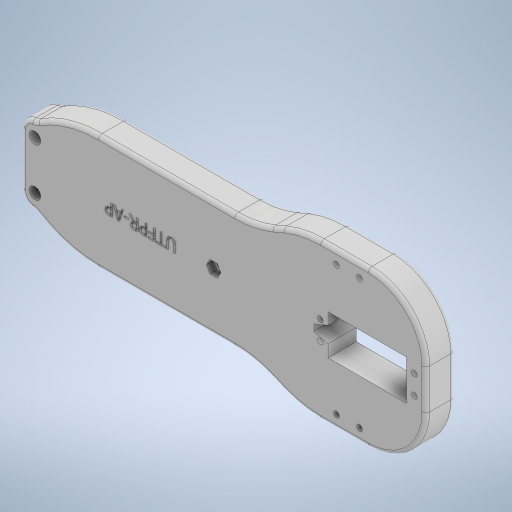
# Autodesk Inventor part: Corpo
Saved by Autodesk Inventor 2024.1 (Build 281209000, 209)
## iProperties
Created: 2024-11-07
Part Number: Corpo
Material: Genérico
Document SubType Name: Modeling
Designer: dimit
Density: 1 g/cm^3
Appearance: Padrão
Author: dimit
Autodesk Inventor part; units mm, degrees
ref_plane "YZ Plane" through (0, 0, 0) normal (1, 0, 0) x (0, 1, 0)
ref_plane "XZ Plane" through (0, 0, 0) normal (0, 1, 0) x (-1, 0, 0)
ref_plane "XY Plane" through (0, 0, 0) normal (0, 0, 1) x (1, 0, 0)
sketch "Esboço1" plane through (0, 0, 0) normal (0, 0, 1) x (1, 0, 0)
  line L0 (44.0084, -10.3855) -> (3.1399, -10.3855)
  line L1 (3.1399, -10.3855) -> (3.1399, 10.3339)
  line L2 (3.1399, 10.3339) -> (44.0084, 10.3339)
  line L3 (44.0084, 10.3339) -> (44.0084, -10.3855)
  line L4 (3.1399, -3.9571) -> (-0.3989, -3.0305)
  line L5 (-0.3989, -3.0305) -> (-1.7282, -2.0962)
  line L6 (-1.7282, -2.0962) -> (-1.7282, 2.1181)
  line L7 (-1.7282, 2.1181) -> (0.2728, 3.0795)
  line L8 (0.2728, 3.0795) -> (3.1399, 4.3343)
  arc A0 (-2.1758, -6.5758) -> (-2.0383, -3.326) centre (-0.9442, -5.0001) ccw
  circle A1 centre (-0.9442, -5.0001) radius 1.9999
  arc A2 (-1.7945, 3.19) -> (0.8219, 4.0617) centre (-0.9442, 5.0002) ccw
  circle A3 centre (-0.9442, 5.0002) radius 2
  arc A4 (46.0562, 5.0474) -> (49.3616, 3.4857) centre (48.0575, 5.0043) ccw
  circle A5 centre (48.0575, 5.0043) radius 2.0017
  arc A6 (48.3945, -3.0289) -> (46.5433, -6.3084) centre (48.0557, -4.9999) ccw
  circle A7 centre (48.0557, -4.9999) radius 1.9999
  line L9 (44.0084, -10.3855) -> (44.0084, -40.3855)
  line L10 (44.0084, 10.3339) -> (44.0084, 40.3339)
  line L11 (44.0084, 40.3339) -> (54.0084, 40.3339)
  line L12 (54.0084, 40.3339) -> (54.0084, -40.3855)
  line L13 (54.0084, -40.3855) -> (44.0084, -40.3855)
  line L14 (-105.4392, -0.0258) -> (-145.4392, -0.0258)
  line L15 (-145.4392, -0.0258) -> (-145.4392, -30.0258)
  line L16 (-145.4392, -30.0258) -> (-145.4392, 29.9742)
  line L17 (-145.4392, 29.9742) -> (-35.4392, 29.9742)
  line L18 (44.0084, 40.3339) -> (-10.9916, 40.3339)
  line L19 (-10.9916, 40.3339) -> (-35.4392, 29.9742)
  line L20 (44.0084, -40.3855) -> (-10.9916, -40.3855)
  line L21 (-145.4392, -30.0258) -> (-35.4392, -30.0258)
  line L22 (-35.4392, -30.0258) -> (-10.9916, -40.3855)
  point P0 (0, 0)
  point P1 (48.3945, -3.0289)
  point P2 (-2.1758, -6.5758)
  point P3 (-2.0383, -3.326)
  point P4 (0.8219, 4.0617)
  dimension "d0" = 2
  dimension "d1" = 30
  dimension "d2" = 30
  dimension "d3" = 10
  dimension "d4" = 40
  dimension "d5" = 30
  dimension "d6" = 60
  dimension "d7" = 110
  dimension "d8" = 55
  dimension "d9" = 55
  dimension "d10" = 110
  constraints: 46 end point, 8 centre point, 8 point on circle, 7 perpendicular, 4 coincident, 3 concentric, 3 parallel, 3 point on line, 3 vertical, 2 horizontal
  measures "d0" radius of A2
  measures "d1" distance of L0.start L9.end
  measures "d2" distance of L2.end L10.end
  measures "d3" distance of L10.end L11.end
  measures "d4" distance of L14.start L14.end
  measures "d5" distance of L14.end L15.end
  measures "d6" distance of L15.end L16.end
  measures "d7" distance of L16.end L17.end
  measures "d8" distance of L10.end L18.end
  measures "d9" distance of L9.end L20.end
  measures "d10" distance of L15.end L21.end
extrude "Extrusão1" add sketch "Esboço1" along normal blind 15 contours L9 L20 L22 L21 L15 L16 L17 L19 L18 L10 L2 L1 L8 L7 L6 L5 L4 L0 | L3 L10 L11 L12 L13 L9
sketch "Esboço2" plane through (0, 0, 0) normal (0, 0, -1) x (-1, 0, 0)
  arc A0 (55.4511, 0.107) -> (57.4146, -0.2455) centre (56.4459, 0.0034) ccw
  circle A1 centre (56.4459, 0.0034) radius 1.0002
  circle A2 centre (56.4459, 0.0034) radius 10
  point P0 (0, 0)
  point P1 (57.4146, -0.2455)
  point P2 (55.4511, 0.107)
  dimension "d13" = 20
  constraints: 3 centre point, 2 coincident, 2 point on circle, 1 concentric
  measures "d13" diameter of A2
extrude "Extrusão2" add sketch "Esboço2" along normal blind 11.5
sketch "Esboço3" plane through (-56.4459, 0.0034, -11.5) normal (0, 0, -1) x (-1, 0, 0)
  circle A0 centre (0, 0) radius 1.0002
  point P0 (-56.4459, -0.0034)
  constraints: 1 centre point
extrude "Extrusão3" cut sketch "Esboço3" against normal blind 30
sketch "Esboço4" plane through (0, 0, 0) normal (0, 0, -1) x (-1, 0, 0)
  arc A0 (121.3485, 15.4476) -> (117.6159, 15.7919) centre (119.4181, 14.9246) ccw
  circle A1 centre (119.4181, 14.9246) radius 2
  line L0 (119.4181, 14.9246) -> (129.4181, 14.9246)
  circle A2 centre (129.4181, 14.9246) radius 2
  point P0 (0, 0)
  dimension "d20" = 2
  dimension "d21" = 10
  dimension "d22" = 4
  constraints: 3 centre point, 2 coincident, 2 end point, 2 point on circle, 1 concentric, 1 horizontal
  measures "d20" radius of A0
  measures "d21" distance of L0.start L0.end
  measures "d22" diameter of A2
extrude "Extrusão4" cut sketch "Esboço4" against normal blind 30
sketch "Esboço5" plane through (0, 0, 0) normal (0, 0, -1) x (-1, 0, 0)
  arc A0 (120.6635, -13.445) -> (117.4381, -15.0358) centre (119.4381, -15.0256) ccw
  circle A1 centre (119.4381, -15.0256) radius 2
  line L0 (119.4381, -15.0256) -> (129.4381, -15.0256)
  circle A2 centre (129.4381, -15.0256) radius 2
  point P0 (0, 0)
  point P1 (120.6635, -13.445)
  dimension "d25" = 2
  dimension "d26" = 10
  dimension "d27" = 4
  constraints: 3 centre point, 2 coincident, 2 end point, 2 point on circle, 1 concentric, 1 horizontal
  measures "d25" radius of A0
  measures "d26" distance of L0.start L0.end
  measures "d27" diameter of A2
extrude "Extrusão5" cut sketch "Esboço5" against normal blind 30
fillet "Arredondamento3" radius 2 4 edges at (-118.2127, -16.6062, 15) (-127.4381, -15.0256, 15) (-127.4181, 14.9246, 15) (-117.4876, 14.4017, 15)
sketch "Esboço8" plane through (0, 0, 0) normal (0, 0, -1) x (-1, 0, 0)
  circle A0 centre (56.4459, 0.0034) radius 1.0002 projected
  line L0 (56.4459, 0.0034) -> (136.4459, 0.0034)
  line L1 (136.4459, 0.0034) -> (136.4459, 20.0034)
  line L2 (136.4459, 20.0034) -> (156.4459, 20.0034)
  line L3 (156.4459, 20.0034) -> (156.4459, -19.9966)
  line L4 (156.4459, -19.9966) -> (136.4459, -19.9966)
  line L5 (136.4459, -19.9966) -> (136.4459, 0.0034)
  point P0 (0, 0)
  dimension "d36" = 80
  dimension "d37" = 20
  dimension "d38" = 20
  dimension "d39" = 40
  dimension "d40" = 20
  constraints: 12 end point, 3 perpendicular, 1 horizontal, 1 point on line
  measures "d36" distance of L0.start L0.end
  measures "d37" distance of L0.end L1.end
  measures "d38" distance of L1.end L2.end
  measures "d39" distance of L2.end L3.end
  measures "d40" distance of L3.end L4.end
extrude "Extrusão6" add sketch "Esboço8" against normal blind 15 contours L1 L2 L3 L4 L5
sketch "Esboço9" plane through (0, 0, 0) normal (0, 0, -1) x (-1, 0, 0)
  circle A0 centre (129.4181, 14.9246) radius 2 projected
  line L0 (129.4181, 14.9246) -> (156.4459, 14.9246)
  line L1 (156.4459, -19.9966) -> (156.4459, 20.0034) projected
  line L2 (156.4459, 14.9246) -> (151.4459, 14.9246)
  line L3 (151.4459, 14.9246) -> (141.4459, 14.9246)
  circle A1 centre (141.4459, 14.9246) radius 1.25
  circle A2 centre (151.4459, 14.9246) radius 1.25
  circle A3 centre (129.4381, -15.0256) radius 2 projected
  line L4 (129.4381, -15.0256) -> (156.4459, -15.0256)
  line L5 (156.4459, -15.0256) -> (151.4459, -15.0256)
  line L6 (151.4459, -15.0256) -> (141.4459, -15.0256)
  circle A4 centre (141.4459, -15.0256) radius 1.25
  circle A5 centre (151.4459, -15.0256) radius 1.25
  point P0 (0, 0)
  dimension "d43" = 5
  dimension "d44" = 10
  dimension "d45" = 2.5
  dimension "d46" = 2.5
  dimension "d47" = 5
  dimension "d48" = 10
  dimension "d49" = 2.5
  dimension "d50" = 2.5
  constraints: 12 end point, 6 point on line, 4 centre point, 4 coincident, 2 horizontal
  measures "d43" distance of L0.end L2.end
  measures "d44" distance of L2.end L3.end
  measures "d45" diameter of A1
  measures "d46" diameter of A2
  measures "d47" distance of L4.end L5.end
  measures "d48" distance of L5.end L6.end
  measures "d49" diameter of A4
  measures "d50" diameter of A5
extrude "Extrusão7" cut sketch "Esboço9" against normal blind 15 contours L0 A1 | L0 A1 | L0 A2 | L0 A2 | L4 A4 | L4 A4 | L4 A5 | L4 A5
sketch "Esboço10" plane through (0, 0, 0) normal (0, 0, -1) x (-1, 0, 0)
  line L0 (109.478, 20.6941) -> (134.736, 20.6941)
  line L1 (134.736, 20.6941) -> (134.736, -21.6092)
  line L2 (134.736, -21.6092) -> (109.478, -21.6092)
  line L3 (109.478, -21.6092) -> (109.478, 20.6941)
  point P0 (0, 0)
  constraints: 8 end point, 2 parallel, 1 horizontal, 1 perpendicular
extrude "Extrusão8" add sketch "Esboço10" against normal blind 15
fillet "Arredondamento5" radius 6 4 edges at (-145.4392, 20.0034, 7.5) (-156.4459, 20.0034, 7.5) (-156.4459, -19.9966, 7.5) (-145.4392, -19.9966, 7.5)
fillet "Arredondamento6" radius 60 2 edges at (-145.4392, 29.9742, 7.5) (-145.4392, -30.0258, 7.5)
fillet "Arredondamento7" radius 30 2 edges at (54.0084, -40.3855, 7.5) (54.0084, 40.3339, 7.5)
fillet "Arredondamento8" radius 50 4 edges at (-35.4392, 29.9742, 7.5) (-10.9916, 40.3339, 7.5) (-10.9916, -40.3855, 7.5) (-35.4392, -30.0258, 7.5)
sketch "Esboço11" plane through (0, 0, 15) normal (0, 0, 1) x (1, 0, 0)
  line L0 (-75.9175, -3.2034) -> (-113.2293, -3.2034) construction
  line L1 (-113.2293, -3.2034) -> (-113.2293, 3.0251) construction
  line L2 (-113.2293, 3.0251) -> (-75.9175, 3.0251) construction
  line L3 (-75.9175, 3.0251) -> (-75.9175, -3.2034) construction
  spline S0 degree 2 poles (-78.6659, 3.0251) (-78.1271, 3.0251) (-77.3263, 2.7433) (-77.0445, 2.4616) knots 0 0 0 1 2 2 2
  spline S1 degree 2 poles (-77.0445, 2.4616) (-76.7232, 2.1452) (-76.4612, 1.2554) (-76.4612, 0.6029) knots 0 0 0 1 2 2 2
  line L4 (-76.4612, 0.6029) -> (-76.4612, -3.2034)
  line L5 (-76.4612, -3.2034) -> (-77.2719, -3.2034)
  line L6 (-77.2719, -3.2034) -> (-77.2719, 0.6029)
  spline S2 degree 2 poles (-77.2719, 0.6029) (-77.2719, 1.028) (-77.3807, 1.6014) (-77.5339, 1.8338) knots 0 0 0 1 2 2 2
  spline S3 degree 2 poles (-77.5339, 1.8338) (-77.6971, 2.0809) (-78.2606, 2.333) (-78.6659, 2.333) knots 0 0 0 1 2 2 2
  spline S4 degree 2 poles (-78.6659, 2.333) (-79.0466, 2.333) (-79.6398, 2.0809) (-79.8029, 1.8338) knots 0 0 0 1 2 2 2
  spline S5 degree 2 poles (-79.8029, 1.8338) (-79.9561, 1.6014) (-80.0649, 1.033) (-80.0649, 0.6227) knots 0 0 0 1 2 2 2
  line L7 (-80.0649, 0.6227) -> (-80.0649, -3.2034)
  line L8 (-80.0649, -3.2034) -> (-80.8756, -3.2034)
  line L9 (-80.8756, -3.2034) -> (-80.8756, 0.6029)
  spline S6 degree 2 poles (-80.8756, 0.6029) (-80.8756, 1.2406) (-80.6185, 2.1501) (-80.2923, 2.4616) knots 0 0 0 1 2 2 2
  spline S7 degree 2 poles (-80.2923, 2.4616) (-80.0006, 2.7483) (-79.2295, 3.0251) (-78.6659, 3.0251) knots 0 0 0 1 2 2 2
  line L10 (-83.4609, 2.8966) -> (-83.4609, -2.4817)
  line L11 (-83.4609, -2.4817) -> (-81.4144, -2.4817)
  line L12 (-81.4144, -2.4817) -> (-81.4144, -3.2034)
  line L13 (-81.4144, -3.2034) -> (-86.3181, -3.2034)
  line L14 (-86.3181, -3.2034) -> (-86.3181, -2.4817)
  line L15 (-86.3181, -2.4817) -> (-84.2716, -2.4817)
  line L16 (-84.2716, -2.4817) -> (-84.2716, 2.8966)
  line L17 (-84.2716, 2.8966) -> (-83.4609, 2.8966)
  line L18 (-90.5842, -2.4817) -> (-87.7467, -2.4817)
  line L19 (-87.7467, -2.4817) -> (-87.7467, -0.7615)
  line L20 (-87.7467, -0.7615) -> (-90.4655, -0.7615)
  line L21 (-90.4655, -0.7615) -> (-90.4655, -0.0397)
  line L22 (-90.4655, -0.0397) -> (-87.7467, -0.0397)
  line L23 (-87.7467, -0.0397) -> (-87.7467, 2.8966)
  line L24 (-87.7467, 2.8966) -> (-86.936, 2.8966)
  line L25 (-86.936, 2.8966) -> (-86.936, -3.2034)
  line L26 (-86.936, -3.2034) -> (-90.5842, -3.2034)
  line L27 (-90.5842, -3.2034) -> (-90.5842, -2.4817)
  spline S8 degree 2 poles (-95.1666, -1.3645) (-95.1666, -0.9691) (-94.8848, -0.2572) (-94.6327, -0.0101) knots 0 0 0 1 2 2 2
  spline S9 degree 2 poles (-94.6327, -0.0101) (-94.3163, 0.3014) (-93.4612, 0.6227) (-92.8086, 0.6227) knots 0 0 0 1 2 2 2
  line L28 (-92.8086, 0.6227) -> (-92.1215, 0.6227)
  line L29 (-92.1215, 0.6227) -> (-92.1215, 2.8966)
  line L30 (-92.1215, 2.8966) -> (-91.3108, 2.8966)
  line L31 (-91.3108, 2.8966) -> (-91.3108, -3.2034)
  line L32 (-91.3108, -3.2034) -> (-92.8432, -3.2034)
  spline S10 degree 2 poles (-92.8432, -3.2034) (-93.387, -3.2034) (-94.1483, -3.0255) (-94.4399, -2.8228) knots 0 0 0 1 2 2 2
  spline S11 degree 2 poles (-94.4399, -2.8228) (-94.781, -2.5905) (-95.1666, -1.8737) (-95.1666, -1.3645) knots 0 0 0 1 2 2 2
  spline S12 degree 2 poles (-94.3213, -1.3398) (-94.3213, -1.6562) (-94.1038, -2.1209) (-93.8813, -2.2692) knots 0 0 0 1 2 2 2
  spline S13 degree 2 poles (-93.8813, -2.2692) (-93.6885, -2.3977) (-93.1744, -2.5015) (-92.7938, -2.5015) knots 0 0 0 1 2 2 2
  line L33 (-92.7938, -2.5015) -> (-92.1215, -2.5015)
  line L34 (-92.1215, -2.5015) -> (-92.1215, -0.0694)
  line L35 (-92.1215, -0.0694) -> (-92.6752, -0.0694)
  spline S14 degree 2 poles (-92.6752, -0.0694) (-93.1695, -0.0694) (-93.7775, -0.2276) (-93.9753, -0.4352) knots 0 0 0 1 2 2 2
  spline S15 degree 2 poles (-93.9753, -0.4352) (-94.1582, -0.6181) (-94.3213, -1.0482) (-94.3213, -1.3398) knots 0 0 0 1 2 2 2
  line L36 (-100.6586, 2.8966) -> (-99.6056, 2.8966)
  line L37 (-99.6056, 2.8966) -> (-97.6778, 0.4694)
  line L38 (-97.6778, 0.4694) -> (-96.7484, 0.4694)
  line L39 (-96.7484, 0.4694) -> (-96.7484, 2.8966)
  line L40 (-96.7484, 2.8966) -> (-95.9377, 2.8966)
  line L41 (-95.9377, 2.8966) -> (-95.9377, -3.2034)
  line L42 (-95.9377, -3.2034) -> (-97.5097, -3.2034)
  spline S16 degree 2 poles (-97.5097, -3.2034) (-98.0337, -3.2034) (-98.7406, -3.0897) (-99.0619, -2.8821) knots 0 0 0 1 2 2 2
  spline S17 degree 2 poles (-99.0619, -2.8821) (-99.3832, -2.6745) (-99.7539, -2.0269) (-99.7539, -1.5474) knots 0 0 0 1 2 2 2
  spline S18 degree 2 poles (-99.7539, -1.5474) (-99.7539, -0.8801) (-99.0718, 0.0245) (-98.4885, 0.242) knots 0 0 0 1 2 2 2
  line L43 (-98.4885, 0.242) -> (-100.6586, 2.8966)
  spline S19 degree 2 poles (-98.9086, -1.4832) (-98.9086, -1.7501) (-98.7208, -2.1604) (-98.5231, -2.2939) knots 0 0 0 1 2 2 2
  spline S20 degree 2 poles (-98.5231, -2.2939) (-98.3501, -2.4076) (-97.8903, -2.5015) (-97.5542, -2.5015) knots 0 0 0 1 2 2 2
  line L44 (-97.5542, -2.5015) -> (-96.7484, -2.5015)
  line L45 (-96.7484, -2.5015) -> (-96.7484, -0.2078)
  line L46 (-96.7484, -0.2078) -> (-97.4603, -0.2078)
  spline S21 degree 2 poles (-97.4603, -0.2078) (-97.8112, -0.2078) (-98.3698, -0.3314) (-98.5626, -0.5242) knots 0 0 0 1 2 2 2
  spline S22 degree 2 poles (-98.5626, -0.5242) (-98.7406, -0.6922) (-98.9086, -1.1668) (-98.9086, -1.4832) knots 0 0 0 1 2 2 2
  line L47 (-103.2043, 0.5979) -> (-100.8958, 0.5979)
  line L48 (-100.8958, 0.5979) -> (-100.8958, -0.1435)
  line L49 (-100.8958, -0.1435) -> (-103.2043, -0.1435)
  line L50 (-103.2043, -0.1435) -> (-103.2043, 0.5979)
  line L51 (-103.5306, 2.8966) -> (-105.587, -3.2034)
  line L52 (-105.587, -3.2034) -> (-106.5855, -3.2034)
  line L53 (-106.5855, -3.2034) -> (-108.6419, 2.8966)
  line L54 (-108.6419, 2.8966) -> (-107.7868, 2.8966)
  line L55 (-107.7868, 2.8966) -> (-107.2331, 1.1911)
  line L56 (-107.2331, 1.1911) -> (-104.9048, 1.1911)
  line L57 (-104.9048, 1.1911) -> (-104.3512, 2.8966)
  line L58 (-104.3512, 2.8966) -> (-103.5306, 2.8966)
  line L59 (-107.0107, 0.4991) -> (-106.0665, -2.373)
  line L60 (-106.0665, -2.373) -> (-105.1273, 0.4991)
  line L61 (-105.1273, 0.4991) -> (-107.0107, 0.4991)
  spline S23 degree 2 poles (-113.0761, -1.3645) (-113.0761, -0.9691) (-112.7943, -0.2572) (-112.5422, -0.0101) knots 0 0 0 1 2 2 2
  spline S24 degree 2 poles (-112.5422, -0.0101) (-112.2258, 0.3014) (-111.3706, 0.6227) (-110.7181, 0.6227) knots 0 0 0 1 2 2 2
  line L62 (-110.7181, 0.6227) -> (-110.031, 0.6227)
  line L63 (-110.031, 0.6227) -> (-110.031, 2.8966)
  line L64 (-110.031, 2.8966) -> (-109.2203, 2.8966)
  line L65 (-109.2203, 2.8966) -> (-109.2203, -3.2034)
  line L66 (-109.2203, -3.2034) -> (-110.7527, -3.2034)
  spline S25 degree 2 poles (-110.7527, -3.2034) (-111.2965, -3.2034) (-112.0578, -3.0255) (-112.3494, -2.8228) knots 0 0 0 1 2 2 2
  spline S26 degree 2 poles (-112.3494, -2.8228) (-112.6905, -2.5905) (-113.0761, -1.8737) (-113.0761, -1.3645) knots 0 0 0 1 2 2 2
  spline S27 degree 2 poles (-112.2308, -1.3398) (-112.2308, -1.6562) (-112.0133, -2.1209) (-111.7908, -2.2692) knots 0 0 0 1 2 2 2
  spline S28 degree 2 poles (-111.7908, -2.2692) (-111.598, -2.3977) (-111.0839, -2.5015) (-110.7033, -2.5015) knots 0 0 0 1 2 2 2
  line L67 (-110.7033, -2.5015) -> (-110.031, -2.5015)
  line L68 (-110.031, -2.5015) -> (-110.031, -0.0694)
  line L69 (-110.031, -0.0694) -> (-110.5847, -0.0694)
  spline S29 degree 2 poles (-110.5847, -0.0694) (-111.079, -0.0694) (-111.687, -0.2276) (-111.8847, -0.4352) knots 0 0 0 1 2 2 2
  spline S30 degree 2 poles (-111.8847, -0.4352) (-112.0676, -0.6181) (-112.2308, -1.0482) (-112.2308, -1.3398) knots 0 0 0 1 2 2 2
  point P0 (0, 0)
  constraints: 2 other
extrude "Extrusão9" cut sketch "Esboço11" against normal blind 2
sketch "Esboço13" plane through (0, 0, 0) normal (0, 0, -1) x (-1, 0, 0)
  arc A0 (-8.9962, -33.7138) -> (-6.0214, -33.7013) centre (-7.5085, -33.7804) ccw
  circle A1 centre (-7.5085, -33.7804) radius 1.4892
  line L0 (-7.5085, -33.7804) -> (-19.5085, -33.7804)
  circle A2 centre (-19.5085, -33.7804) radius 1.5
  arc A3 (-6.6764, 35.0879) -> (-8.1018, 35.214) centre (-7.5067, 33.8217) ccw
  circle A4 centre (-7.5067, 33.8217) radius 1.5141
  line L1 (-7.5067, 33.8217) -> (-19.5067, 33.8217)
  circle A5 centre (-19.5067, 33.8217) radius 1.5
  point P0 (0, 0)
  dimension "d62" = 12
  dimension "d63" = 3
  dimension "d64" = 12
  dimension "d65" = 3
  constraints: 6 centre point, 4 coincident, 4 end point, 4 point on circle, 2 concentric, 2 horizontal
  measures "d62" distance of L0.start L0.end
  measures "d63" diameter of A2
  measures "d64" distance of L1.start L1.end
  measures "d65" diameter of A5
extrude "Extrusão10" cut sketch "Esboço13" against normal blind 20
sketch "Esboço14" plane through (0, 0, 15) normal (0, 0, 1) x (1, 0, 0)
  circle A0 centre (-0.9442, -5.0001) radius 1.9999 projected
  circle A1 centre (-0.9442, -5.0001) radius 1.9999
  circle A2 centre (-0.9442, 5.0002) radius 2 projected
  circle A3 centre (-0.9442, 5.0002) radius 2
  circle A4 centre (48.0575, 5.0043) radius 2.0017 projected
  circle A5 centre (48.0575, 5.0043) radius 2.0017
  circle A6 centre (48.0557, -4.9999) radius 1.9999 projected
  circle A7 centre (48.0557, -4.9999) radius 1.9999
  circle A8 centre (48.0557, -4.9999) radius 1.5
  circle A9 centre (48.0575, 5.0043) radius 1.5
  circle A10 centre (-0.9442, 5.0002) radius 1.5
  circle A11 centre (-0.9442, -5.0001) radius 1.5
  point P0 (0, 0)
  dimension "d68" = 3
  dimension "d69" = 3
  dimension "d70" = 3
  dimension "d71" = 3
  constraints: 8 centre point, 8 coincident
  measures "d68" diameter of A8
  measures "d69" diameter of A9
  measures "d70" diameter of A10
  measures "d71" diameter of A11
extrude "Extrusão11" add sketch "Esboço14" against normal up to surface (15 mm away)
sketch "Esboço15" plane through (-56.4459, 0.0034, -11.5) normal (0, 0, -1) x (-1, 0, 0)
  circle A0 centre (0, 0) radius 7.5
  circle A1 centre (0, 0) radius 1.0002 projected
  circle A2 centre (0, 0) radius 15.3264
  point P0 (-56.4459, -0.0034)
  dimension "d76" = 15
  constraints: 2 centre point, 1 coincident
  measures "d76" diameter of A0
extrude "Extrusão12" cut sketch "Esboço15" against normal up to surface (11.5 mm away) contours A2
sketch "Esboço16" plane through (-56.4459, 0.0034, -11.5) normal (0, 0, -1) x (-1, 0, 0)
  circle A0 centre (0, 0) radius 1.0002
  circle A1 centre (0, 0) radius 7.5
  point P0 (-56.4459, -0.0034)
  constraints: 2 centre point, 1 coincident
extrude "Extrusão13" add sketch "Esboço16" along normal blind 2
fillet "Arredondamento11" radius 18 1 edges at (-48.9459, 0.0034, 0)
sketch "Esboço17" plane through (-56.4459, 0.0034, -13.5) normal (0, 0, -1) x (-1, 0, 0)
  circle A0 centre (0, 0) radius 4.75
  circle A1 centre (0, 0) radius 1.0002
  point P0 (-56.4459, -0.0034)
  dimension "d82" = 9.5
  constraints: 2 centre point, 1 coincident
  measures "d82" diameter of A0
extrude "Extrusão14" add sketch "Esboço17" along normal blind 5
fillet "Arredondamento12" radius 1 1 edges at (-51.6959, 0.0034, -18.5)
sketch "Esboço18" plane through (-56.4459, 0.0034, -18.5) normal (0, 0, -1) x (-1, 0, 0)
  circle A0 centre (0, 0) radius 2
  point P0 (-56.4459, -0.0034)
  dimension "d86" = 4
  constraints: 1 centre point
  measures "d86" diameter of A0
extrude "Extrusão15" cut sketch "Esboço18" against normal blind 50
sketch "Esboço19" plane through (0, 0, 15) normal (0, 0, 1) x (1, 0, 0)
  circle A0 centre (-56.4459, 0.0034) radius 3.75 projected
  line L0 (-56.4459, 0.0034) -> (-56.4459, -3.4966)
  line L1 (-56.4459, -3.4966) -> (-56.4459, 3.5034)
  circle A1 centre (-56.4459, 0.0034) radius 4.75 projected
  line L2 (-56.4459, 3.5034) -> (-56.4459, 0.0034)
  line L3 (-56.4459, 0.0034) -> (-52.9459, 0.0034)
  line L4 (-52.9459, 0.0034) -> (-59.9459, 0.0034)
  circle A2 centre (-56.4459, 0.0034) radius 3.5
  line L5 (-59.9459, 0.0034) -> (-56.4108, 0.0034) construction
  line L6 (-59.9459, 0.0034) -> (-58.1959, 3.0345)
  line L7 (-58.1959, -3.0277) -> (-59.9459, 0.0034)
  line L8 (-52.9459, 0.0034) -> (-54.6959, 3.0345)
  line L9 (-54.6959, -3.0277) -> (-52.9459, 0.0034)
  line L10 (-54.6959, 3.0345) -> (-58.1959, 3.0345)
  line L11 (-54.6959, -3.0277) -> (-58.1959, -3.0277)
  line L12 (-52.7727, -0.0966) -> (-54.5804, -3.2277)
  line L13 (-54.5804, -3.2277) -> (-58.3113, -3.2277)
  line L14 (-58.3113, -3.2277) -> (-60.1191, -0.0966)
  line L15 (-52.7727, 0.1034) -> (-54.5804, 3.2345)
  line L16 (-54.5804, 3.2345) -> (-58.1959, 3.2345)
  line L17 (-60.1191, 0.1034) -> (-58.3691, 3.1345)
  line L18 (-52.7727, 0.1034) -> (-52.7727, -0.0966)
  line L19 (-58.3691, 3.1345) -> (-58.1959, 3.2345)
  line L20 (-60.1191, -0.0966) -> (-60.1191, 0.1034)
  point P0 (0, 0)
  dimension "d89" = 3.5
  dimension "d90" = 7
  dimension "d91" = 3.5
  dimension "d92" = 7
  dimension "d94" = 3.5
  dimension "d95" = 3.5
  dimension "d96" = 3.5
  dimension "d97" = 3.5
  dimension "d98" = 0.2
  dimension "d99" = 0.2
  dimension "d100" = 0.2
  constraints: 42 end point, 6 point on circle, 3 horizontal, 2 parallel, 2 point on line, 2 vertical, 1 centre point, 1 coincident, 1 collinear, 3 other
  measures "d89" distance of L0.start L0.end
  measures "d90" distance of L0.end L1.end
  measures "d91" distance of L2.end L3.end
  measures "d92" distance of L3.end L4.end
  measures "d94" distance of L4.end L6.end
  measures "d95" distance of L4.end L7.start
  measures "d96" distance of L3.end L8.end
  measures "d97" distance of L3.end L9.start
  measures "d98" distance between parallel lines of L9 L12
  measures "d99" distance between parallel lines of L8 L15
  measures "d100" distance between parallel lines of L6 L17
extrude "Extrusão16" cut sketch "Esboço19" against normal blind 3.5 contours L3 L9 L11 L0 | L4 L6 L10 L1 | L1 L10 L8 L3 | L0 L11 L7 L4 | L11 A2 L13 L0 | L0 L13 A2 L11 | L10 A2 L16 L1 | L1 L16 A2 L10 | L8 A2 L15 | A2 L15 L18 L12 | A2 L12 L9 | A2 L14 L20 L17 | L7 A2 L14 | A2 L17 L6 | A2 L12 L13 | A2 L13 L14 | A2 L16 L15 | A2 L17 L19 L16
sketch "Esboço20" plane through (0, 0, 15) normal (0, 0, 1) x (1, 0, 0)
  line L0 (-137.8499, -17.2521) -> (-153.5171, -17.2521)
  line L1 (-153.5171, -17.2521) -> (-153.5171, 17.6377)
  line L2 (-153.5171, 17.6377) -> (-137.8499, 17.6377)
  line L3 (-137.8499, 17.6377) -> (-137.8499, -17.2521)
  point P0 (0, 0)
  constraints: 8 end point, 2 parallel, 1 horizontal, 1 perpendicular
extrude "Extrusão17" add sketch "Esboço20" against normal up to surface (15 mm away)
sketch "Esboço21" plane through (0, 0, 15) normal (0, 0, 1) x (1, 0, 0)
  circle A0 centre (-149.5725, -12.4544) radius 3
  line L0 (-149.5725, -12.4544) -> (-149.5725, 20.3011)
  arc A1 (-150.9425, 20.024) -> (-148.2681, 20.9098) centre (-151.4392, 26.0034) ccw projected
  line L1 (-149.5725, 20.3011) -> (-149.5725, 12.5011)
  circle A2 centre (-149.5725, 12.5011) radius 3
  point P0 (0, 0)
  dimension "d105" = 6
  dimension "d106" = 7.8
  constraints: 4 end point, 2 centre point, 1 coincident, 1 point on circle, 1 point on line, 1 vertical
  measures "d105" diameter of A0
  measures "d106" distance of L0.end L1.end
extrude "Extrusão18" cut sketch "Esboço21" against normal up to surface (15 mm away)
fillet "Arredondamento13" radius 2 40 edges at (-133.0478, 27.6636, 0) (-149.5526, 20.3077, 0) (-154.8606, 18.1078, 0) (-156.4459, 0.024, 0) (-154.8606, -18.0599, 0) (-149.5445, -20.2624, 0) (-132.9706, -27.6917, 0) (-80.9969, -30.0258, 0) (-35.6424, -31.0265, 0) (-23.2154, -35.2056, 0) (-10.7883, -39.3848, 0) (11.5867, -40.3855, 0) (45.2216, -31.5987, 0) (54.0084, -0.0258, 0) (45.2216, 31.5471, 0) (11.5867, 40.3339, 0) (-10.7883, 39.3332, 0) (-23.2154, 35.154, 0) (-35.6424, 30.9749, 0) (-81.0766, 29.9742, 0) (-133.0478, 27.6636, 15) (-149.5526, 20.3077, 15) (-154.8606, 18.1078, 15) (-156.4459, 0.024, 15) (-154.8606, -18.0599, 15) (-149.5445, -20.2624, 15) (-132.9706, -27.6917, 15) (-80.9969, -30.0258, 15) (-35.6424, -31.0265, 15) (-23.2154, -35.2056, 15) (-10.7883, -39.3848, 15) (11.5867, -40.3855, 15) (45.2216, -31.5987, 15) (54.0084, -0.0258, 15) (45.2216, 31.5471, 15) (11.5867, 40.3339, 15) (-10.7883, 39.3332, 15) (-23.2154, 35.154, 15) (-35.6424, 30.9749, 15) (-81.0766, 29.9742, 15)
sketch "Esboço22" plane through (0, 0, 0) normal (0, 0, -1) x (-1, 0, 0)
  line L0 (-3.1399, -3.9571) -> (0.3989, -3.0305) projected
  line L1 (0.3989, -3.0305) -> (4.2086, -2.033)
  line L2 (4.2086, -2.033) -> (4.2086, 1.2299)
  line L3 (1.7282, 2.1181) -> (-0.2728, 3.0795) projected
  line L4 (4.2086, 1.2299) -> (1.7282, 2.1181)
  line L5 (1.7282, 2.1181) -> (-1.0877, -2.0186)
  line L6 (-1.0877, -2.0186) -> (0.3989, -3.0305)
  point P0 (0, 0)
  constraints: 10 end point, 1 collinear, 1 perpendicular, 1 vertical
extrude "Extrusão19" cut sketch "Esboço22" against normal blind 30
fillet "Arredondamento14" radius 0.5 10 edges at (23.5742, -10.3855, 0) (3.1399, -7.1713, 0) (-0.5344, -2.995, 0) (1.7063, 3.7069, 0) (3.1399, 7.3341, 0) (23.5742, 10.3339, 0) (44.0084, -0.0258, 0) (-2.9684, 1.674, 0) (-0.7277, 2.5988, 0) (-4.2086, -0.4015, 0)
